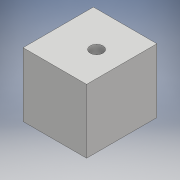
# Autodesk Inventor part: 02BombaJarron
Saved by Autodesk Inventor 2018 (Build 220112000, 112)
## iProperties
Created: 2020-06-23
Part Number: 02BombaJarron
Material: Generic
Document SubType Name: Modeling
Designer: Ivan
Density: 1 g/cm^3
Appearance: Default
Author: Ivan
Autodesk Inventor part; units mm, degrees
ref_plane "YZ Plane" through (0, 0, 0) normal (1, 0, 0) x (0, 1, 0)
ref_plane "XZ Plane" through (0, 0, 0) normal (0, 1, 0) x (-1, 0, 0)
ref_plane "XY Plane" through (0, 0, 0) normal (0, 0, 1) x (1, 0, 0)
sketch "Sketch1" plane through (0, 0, 0) normal (0, 0, 1) x (1, 0, 0)
  circle A0 centre (0, 0) radius 5
  circle A1 centre (0, 0) radius 7
  dimension "d0" = 10
  dimension "d1" = 14
  constraints: 2 centre point, 2 coincident
  measures "d0" diameter of A0
  measures "d1" diameter of A1
extrude "Extrusion1" add sketch "Sketch1" along normal blind 10
sketch "Sketch2" plane through (0, 0, 10) normal (0, 0, 1) x (1, 0, 0)
  line L0 (-30, -27.5) -> (19.666, -27.5)
  line L1 (19.666, -27.5) -> (19.666, 27.5)
  line L2 (19.666, 27.5) -> (-30, 27.5)
  line L3 (-30, 27.5) -> (-30, -27.5)
  point P0 (0, 0)
  point P1 (-30, 0)
  dimension "d4" = 19.666
  dimension "d5" = 55
  dimension "d6" = 30
  constraints: 8 end point, 2 parallel, 1 horizontal, 1 horizontal alignment, 1 midpoint, 1 perpendicular
  measures "d4" distance from line of L1 point (0, 0)
  measures "d5" distance of L2.end L0.start
  measures "d6" distance from line of L3 point (0, 0)
extrude "Extrusion2" add sketch "Sketch2" along normal blind 50
fillet "Fillet1" radius 0.5 1 edges at (-5, 0, 0)
sketch "Sketch3" plane through (0, 0, 10) normal (0, 0, -1) x (-1, 0, 0)
  circle A0 centre (0, 0) radius 5 projected
extrude "Extrusion3" cut sketch "Sketch3" against normal up to surface (50 mm away)
body "Solid1"
